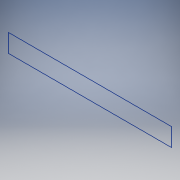
# Autodesk Inventor part: base
Saved by Autodesk Inventor 2018.1 (Build 221171000, 171)
## iProperties
Created: 2017-10-18
Part Number: base
Material: アルミニウム 6061
Document SubType Name: Modeling
Designer: kuwano
Density: 2.7 g/cm^3
Appearance: アルミニウム - フラット
Mass: 1640.25 g
Surface Area: 4140 cm^2
Volume: 607.5 cm^3
Author: kuwano
Autodesk Inventor part; units mm, degrees
ref_plane "YZ Plane" through (0, 0, 0) normal (1, 0, 0) x (0, 1, 0)
ref_plane "XZ Plane" through (0, 0, 0) normal (0, 1, 0) x (-1, 0, 0)
ref_plane "XY Plane" through (0, 0, 0) normal (0, 0, 1) x (1, 0, 0)
sketch "スケッチ1" plane through (0, 0, 0) normal (0, 1, 0) x (-1, 0, 0)
  line L0 (675, 75) -> (-675, 75)
  line L1 (-675, 75) -> (-675, -75)
  line L2 (-675, -75) -> (675, -75)
  line L3 (675, -75) -> (675, 75)
  line L4 (0, -105) -> (0, 105) projected
  line L5 (945, 0) -> (-945, 0) projected
  point P0 (0, 0)
  point P1 (0, -75)
  point P2 (675, 0)
  dimension "d0" = 1350
  dimension "d1" = 150
  constraints: 8 end point, 2 midpoint, 2 parallel, 2 point on line, 1 horizontal, 1 perpendicular
  measures "d0" distance of L0.start L0.end
  measures "d1" distance of L2.end L0.start
extrude "押し出し1" add sketch "スケッチ1" along normal blind 3
